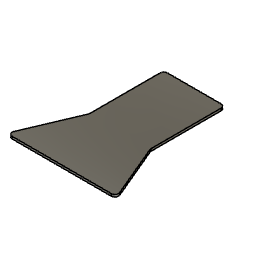
weapon holder v1 (Autodesk Fusion 360 design; units mm, degrees)
Autodesk Fusion 360 part; units mm, degrees
sketch "Sketch1" plane through (0, 0, 0) normal (0, 0, 1) x (1, 0, 0)
  line L0 (-38.481, 0) -> (38.481, 0)
  line L1 (38.481, 0) -> (21.3487, 40.63)
  line L2 (21.3487, 40.63) -> (21.3487, 92.71)
  line L3 (21.3487, 92.71) -> (-21.3487, 92.71)
  line L4 (-21.3487, 92.71) -> (-21.3487, 40.63)
  line L5 (-21.3487, 40.63) -> (-38.481, 0)
  line L6 (-21.3487, 40.63) -> (-21.3487, 0)
  line L7 (21.3487, 40.63) -> (21.3487, 0)
  dimension "d1" = 76.962
  dimension "d3" = 92.71
  dimension "d4" = 44.0944
  dimension "d5" = 42.6974
  constraint horizontal L0
  constraint perpendicular L0 L2
  constraint perpendicular L2 L3
  constraint perpendicular L3 L4
  constraint coincident L0 L6.end
  constraint perpendicular L0 L6
  constraint coincident L0 L7.end
  constraint perpendicular L0 L7
  constraint equal L6 L7
  constraint equal L1 L5
  constraint midpoint origin L0
  measures "d1" distance of L0.start L0.end
  measures "d3" distance of L0 L3
  measures "d4" distance of L0.start L4.end
  measures "d5" distance of L2 L4
extrude "Extrude1" add sketch "Sketch1" along normal blind 1.5748
fillet "Fillet1" radius 2.54 6 edges at (21.3487, 92.71, 0.7874) (-21.3487, 92.71, 0.7874) (-21.3487, 40.63, 0.7874) (-38.481, 0, 0.7874) (21.3487, 40.63, 0.7874) (38.481, 0, 0.7874)
